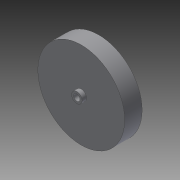
# Autodesk Inventor part: Front Wheel
Saved by Autodesk Inventor 2014 SP1 (Build 180222100, 222)
## iProperties
Created: 2014-01-12
Part Number: Front Wheel
Material: Generic
Document SubType Name: Modeling
Designer: tom
Density: 1 g/cm^3
Appearance: Default
d0: 4.125 in
d1: 0.300 in
d2: 0.500 in
d3: 0.830 in
d4: 0.00 deg
d5: 1.250 in
d6: 0.00 deg
Author: tom
Autodesk Inventor part; units mm, degrees
ref_plane "YZ Plane" through (0, 0, 0) normal (1, 0, 0) x (0, 1, 0)
ref_plane "XZ Plane" through (0, 0, 0) normal (0, 1, 0) x (-1, 0, 0)
ref_plane "XY Plane" through (0, 0, 0) normal (0, 0, 1) x (1, 0, 0)
sketch "Sketch1" plane through (0, 0, 0) normal (0, 0, 1) x (1, 0, 0)
  circle A0 centre (0, 0) radius 52.3875
  circle A1 centre (0, 0) radius 3.81
  circle A2 centre (0, 0) radius 6.35
  dimension "d0" = 104.775
  dimension "d1" = 7.62
  dimension "d2" = 12.7
  constraints: 3 centre point, 3 coincident
  measures "d0" diameter of A0
  measures "d1" diameter of A1
  measures "d2" diameter of A2
extrude "Extrusion1" add sketch "Sketch1" along normal mid plane 21.082 contours A0
extrude "Extrusion2" add sketch "Sketch1" along normal mid plane 31.75 contours A2
body "Solid1"
